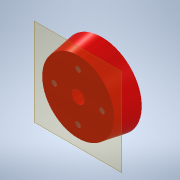
# Autodesk Inventor part: Stator_N5065
Saved by Autodesk Inventor 2021 (Build 250183000, 183)
## iProperties
Created: 2020-08-28
Part Number: Stator_N5065
Material: Generic
Document SubType Name: Modeling
Designer: Hagihara Yuya
Density: 1 g/cm^3
Appearance: 赤
Author: Hagihara Yuya
Autodesk Inventor part; units mm, degrees
ref_plane "YZ Plane" through (0, 0, 0) normal (1, 0, 0) x (0, 1, 0)
ref_plane "XZ Plane" through (0, 0, 0) normal (0, 1, 0) x (-1, 0, 0)
sketch "スケッチ7" plane through (0, 0, 0) normal (0, 0, 1) x (1, 0, 0)
  circle A0 centre (0, 0) radius 25
  dimension "d32" = 50
  constraints: 1 centre point, 1 coincident
  measures "d32" diameter of A0
ref_plane "作業平面7" through (0, 0, 15) normal (0, 0, 1) x (1, 0, 0)
sketch "スケッチ8" plane through (0, 0, 15) normal (0, 0, 1) x (1, 0, 0)
  circle A0 centre (0, 0) radius 22.5
  dimension "d34" = 45
  constraints: 1 centre point, 1 coincident
  measures "d34" diameter of A0
loft "ロフト2" add profiles "スケッチ7", "スケッチ8"
sketch "スケッチ5" plane through (0, 0, 15) normal (0, 0, 1) x (1, 0, 0)
  point P0 (0, 0)
  point P1 (0, 0)
  constraints: 1 coincident
hole "穴1" at (0, 0, 15) direction (0, 0, -1) diameter 8 end through all
sketch "スケッチ6" plane through (0, 0, 15) normal (0, 0, 1) x (1, 0, 0)
  point P0 (0, 0)
  point P1 (15, 0)
  point P2 (0, 15)
  point P3 (-15, 0)
  point P4 (0, -15)
  point P5 (0, 0)
  dimension "d21" = 360
  dimension "d23" = 30
  constraints: 1 coincident, 1 horizontal alignment, 5 other
  measures "d23" distance of point (-15, 0) point (15, 0)
hole "穴2" at (15, 0, 15) at (0, 15, 15) at (-15, 0, 15) at (0, -15, 15) direction (0, 0, -1) diameter 3.4587 depth 10.8 tip angle 118 thread size "M4x0.5" class "6H" standard "ISO Metric profile"
